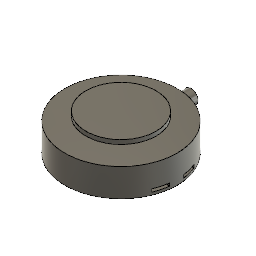
deadbolt-knob-cover (Autodesk Fusion 360 design; units mm, degrees)
Autodesk Fusion 360 part; units mm, degrees
sketch "Sketch1" plane through (0, 0, 0) normal (0, 1, 0) x (1, 0, 0)
  circle A0 centre (0, 0) radius 40
  constraint coincident A0.centre origin
extrude "Extrude1" add sketch "Sketch1" along normal blind 20
sketch "Sketch2" plane through (0, 0, 0) normal (0, -1, 0) x (1, 0, 0)
  circle A0 centre (0, 0) radius 40
  line L0 (8, 20) -> (-8, 20)
  line L1 (-8, 20) -> (-8, -20)
  line L2 (-8, -20) -> (8, -20)
  line L3 (8, -20) -> (8, 20)
  line L4 (8, 20) -> (-8, -20) construction
  line L5 (-8, 20) -> (8, -20) construction
  dimension "d3" = 40
  dimension "d4" = 16
  constraint perpendicular L0 L1
  constraint parallel L0 L2
  constraint parallel L1 L3
  constraint horizontal L0
  constraint coincident L4 A0.centre
  constraint coincident L5 A0.centre
  constraint coincident A0.centre origin
  measures "d3" distance of L0.end L1.end
  measures "d4" distance of L1.end L2.end
extrude "Extrude2" cut sketch "Sketch2" against normal blind 16 contours L0 L1 L2 L3
sketch "Sketch3" plane through (0, 20, 0) normal (0, 1, 0) x (-1, 0, 0)
  circle A0 centre (0, 0) radius 40
  circle A1 centre (0, 0) radius 30
  constraint coincident A0.centre A1.centre
extrude "Extrude3" add sketch "Sketch3" along normal blind 5 draft 10 contours A1
sketch "Sketch4" plane through (0, 25, 0) normal (0, 1, 0) x (-1, 0, 0)
  circle A0 centre (0, 0) radius 30.8816
  circle A1 centre (0, 0) radius 20
  constraint coincident A0.centre A1.centre
extrude "Extrude4" add sketch "Sketch4" along normal blind 5 draft 10 contours A1
sketch "Sketch5" plane through (0, 30, 0) normal (0, 1, 0) x (-1, 0, 0)
  circle A0 centre (0, 0) radius 20.8816
  circle A1 centre (0, 0) radius 10
  constraint coincident A0.centre A1.centre
extrude "Extrude5" add sketch "Sketch5" along normal blind 5 draft 10 contours A1
sketch "Sketch6" plane through (0, 0, -20) normal (0, 0, 1) x (1, 0, 0)
  line L0 (-8, 0) -> (8, 0)
  line L1 (8, 0) -> (8, 16)
  line L2 (8, 16) -> (-8, 16)
  line L3 (-8, 16) -> (-8, 0)
  circle A0 centre (0, 10) radius 5
  dimension "d13" = 10
  measures "d13" diameter of A0
extrude "Extrude6" add sketch "Sketch6" against normal blind 30 contours A0
sketch "Sketch7" plane through (0, 0, 0) normal (0, -1, 0) x (1, 0, 0)
  line L0 (-8, 20) -> (8, 20)
  line L1 (8, 20) -> (8, -20)
  line L2 (8, -20) -> (-8, -20)
  line L3 (-8, -20) -> (-8, 20)
  circle A0 centre (0, 0) radius 40
  line L4 (8, 23) -> (-8, 23)
  line L5 (-8, 23) -> (-8, -23)
  line L6 (-8, -23) -> (8, -23)
  line L7 (8, -23) -> (8, 23)
  line L8 (8, 23) -> (-8, -23) construction
  line L9 (-8, 23) -> (8, -23) construction
  dimension "d16" = 46
  constraint perpendicular L4 L5
  constraint parallel L4 L6
  constraint parallel L5 L7
  constraint horizontal L4
  constraint coincident L8 A0.centre
  constraint coincident L9 A0.centre
  constraint coincident A0.centre origin
  measures "d16" distance of L4.end L5.end
extrude "Extrude7" cut sketch "Sketch7" against normal blind 16 contours L0 L4 L5 L7 | L2 L5 L6 L7
sketch "Sketch8" plane through (-8, 0, 0) normal (1, 0, 0) x (0, 0, -1)
  line L0 (-23, 0) -> (23, 0)
  line L1 (23, 0) -> (23, 16)
  line L2 (23, 16) -> (-23, 16)
  line L3 (-23, 16) -> (-23, 0)
  circle A0 centre (-10, 5) radius 3
  circle A1 centre (10, 5) radius 3
  dimension "d19" = 6
  dimension "d20" = 6
  measures "d19" diameter of A0
  measures "d20" diameter of A1
extrude "Extrude8" add sketch "Sketch8" against normal blind 35 contours A0 | A1
sketch "Sketch9" plane through (8, 0, 0) normal (-1, 0, 0) x (0, 0, 1)
  line L0 (-23, 0) -> (23, 0)
  line L1 (23, 0) -> (23, 16)
  line L2 (23, 16) -> (-23, 16)
  line L3 (-23, 16) -> (-23, 0)
  circle A0 centre (-10, 5) radius 3
  circle A1 centre (10, 5) radius 3
  dimension "d23" = 6
  dimension "d24" = 6
  measures "d23" diameter of A0
  measures "d24" diameter of A1
extrude "Extrude9" add sketch "Sketch9" against normal blind 35 contours A0 | A1
sketch "Sketch10" plane through (0, 16, 0) normal (0, -1, 0) x (1, 0, 0)
  line L0 (8, -23) -> (8, 23)
  line L1 (8, 23) -> (-8, 23)
  line L2 (-8, 23) -> (-8, -23)
  line L3 (-8, -23) -> (8, -23)
  arc A0 (8, 4.6435) -> (3.2947, 23) centre (-30.159, 4.6435) ccw
  spline S0 degree 3 poles (-4.619, -39.7324) (-4.619, -39.7324) (-4.3638, -39.7621) (-3.9791, -39.8041) (-3.092, -39.8828) (-2.5302, -39.9247) (-1.2985, -39.9837) (-0.6285, -40) (0.6285, -40) (1.2985, -39.9837) (2.5302, -39.9247) (3.092, -39.8828) (3.9791, -39.8041) (4.3638, -39.7621) (4.8743, -39.7027) (5, -39.6863) (5, -39.6863) knots 0 0.188556 0.188556 0.188556 0.188556 0.377112 0.377112 0.565667 0.565667 0.754221 0.754221 0.942775 0.942775 1.13133 1.13133 1.319886 1.319886 1.508442 1.508442 1.508442 1.508442
  arc A1 (-3.2947, 23) -> (-8, 4.6435) centre (30.159, 4.6435) ccw
  arc A2 (-8, -4.6435) -> (-3.2947, -23) centre (30.159, -4.6435) ccw
  arc A3 (3.2947, -23) -> (8, -4.6435) centre (-30.159, -4.6435) ccw
  point P0 (-40, 0)
  constraint tangent L0 A0
  constraint coincident L0 A0.start
  constraint coincident L1 A0.end
extrude "Extrude10" add sketch "Sketch10" along normal blind 16 contours L0 L3 A3 | L0 L1 A0 | L2 L3 A2 | L1 L2 A1
sketch "Sketch11" plane through (0, 0, 0) normal (0, -1, 0) x (1, 0, 0)
  line L0 (8, 4.6435) -> (8, -4.6435)
  arc A0 (3.2947, -23) -> (8, -4.6435) centre (-30.159, -4.6435) ccw
  line L1 (3.2947, -23) -> (-3.2947, -23)
  arc A1 (-8, -4.6435) -> (-3.2947, -23) centre (30.159, -4.6435) ccw
  line L2 (-8, -4.6435) -> (-8, 4.6435)
  arc A2 (-3.2947, 23) -> (-8, 4.6435) centre (30.159, 4.6435) ccw
  line L3 (-3.2947, 23) -> (3.2947, 23)
  arc A3 (8, 4.6435) -> (3.2947, 23) centre (-30.159, 4.6435) ccw
  circle A4 centre (0, 0) radius 40
  line L4 (-43, -7) -> (-43, -13)
  line L5 (45, -15) -> (-45, -15)
  line L6 (-45, -5) -> (45, -5)
  line L7 (-43, 13) -> (-43, 7)
  line L8 (45, 5) -> (-45, 5)
  line L9 (-45, 15) -> (45, 15)
  constraint perpendicular L4 L5
  constraint perpendicular L4 L6
  constraint perpendicular L7 L8
  constraint horizontal L9
extrude "Extrude11" cut sketch "Sketch11" along normal blind 2 from surface at -4 contours A3 A4 L8 L9 | A0 A4 L5 L6 | A2 A4 L8 L9 | A1 A4 L5 L6
delete_face "DeleteFace1" 1 faces at (39.8327, 2.5729, -11.7633)
delete_face "DeleteFace2" 1 faces at (39.925, 7.7516, 11.1952)
delete_face "DeleteFace3" 1 faces at (-39.8327, 2.5729, 11.7633)
delete_face "DeleteFace4" 1 faces at (-39.925, 7.7516, -11.1952)
sketch "Sketch12" plane through (0, 0, 0) normal (0, -1, 0) x (1, 0, 0)
  line L0 (8, 4.6435) -> (8, -4.6435)
  arc A0 (3.2947, -23) -> (8, -4.6435) centre (-30.159, -4.6435) ccw
  line L1 (3.2947, -23) -> (-3.2947, -23)
  arc A1 (-8, -4.6435) -> (-3.2947, -23) centre (30.159, -4.6435) ccw
  line L2 (-8, -4.6435) -> (-8, 4.6435)
  arc A2 (-3.2947, 23) -> (-8, 4.6435) centre (30.159, 4.6435) ccw
  line L3 (-3.2947, 23) -> (3.2947, 23)
  arc A3 (8, 4.6435) -> (3.2947, 23) centre (-30.159, 4.6435) ccw
  circle A4 centre (0, 0) radius 40
  circle A5 centre (0, 0) radius 22.5
  dimension "d33" = 45
  constraint coincident A4.centre A5.centre
  measures "d33" diameter of A5
extrude "Extrude12" cut sketch "Sketch12" against normal blind 4 contours L0 A0 A3 A5 | A1 L2 A2 A5
delete_face "DeleteFace5" 1 faces at (-5.2939, 33.3333, -9.1693)
delete_face "DeleteFace6" 1 faces at (-20.5622, 28.3333, -1.0262)
delete_face "DeleteFace7" 1 faces at (-30.5497, 23.3333, -1.5247)
sketch "Sketch13" plane through (0, 20, 0) normal (0, 1, 0) x (-1, 0, 0)
  circle A0 centre (0, 0) radius 40
  circle A1 centre (0, 0) radius 20
  constraint concentric A0 A1
extrude "Extrude13" add sketch "Sketch13" along normal blind 6 contours A1
sketch "Sketch14" plane through (0, 20, 0) normal (0, 1, 0) x (-1, 0, 0)
  circle A0 centre (0, 0) radius 20
  circle A1 centre (0, 0) radius 40
  circle A2 centre (0, 0) radius 25
  constraint coincident A0.centre A1.centre
extrude "Extrude14" add sketch "Sketch14" along normal blind 3 from surface at 3 contours A2
